Autodesk Fusion 360 part; units mm, degrees
(part 5 of 5)
  spline S9 degree 5 poles (1.8021, -146.297) (1.7927, -146.2963) (1.774, -146.2951) (1.746, -146.2934) (1.7087, -146.2912) (1.6621, -146.2888) (1.6156, -146.2866) (1.5692, -146.2847) (1.5229, -146.2831) (1.4766, -146.2818) (1.4305, -146.2807) (1.3844, -146.2799) (1.3384, -146.2794) (1.2924, -146.2792) (1.2466, -146.2792) (1.2009, -146.2795) (1.1552, -146.2801) (1.1097, -146.281) (1.0642, -146.2822) (1.0189, -146.2836) (0.9736, -146.2854) (0.9285, -146.2874) (0.8834, -146.2897) (0.8385, -146.2923) (0.7937, -146.2951) (0.7489, -146.2983) (0.7044, -146.3018) (0.6599, -146.3055) (0.6155, -146.3095) (0.5713, -146.3139) (0.5271, -146.3185) (0.4832, -146.3234) (0.4393, -146.3287) (0.3956, -146.3342) (0.352, -146.3401) (0.3085, -146.3462) (0.2652, -146.3527) (0.222, -146.3594) (0.179, -146.3665) (0.1361, -146.3739) (0.0934, -146.3816) (0.0508, -146.3896) (0.0084, -146.3979) (-0.0338, -146.4066) (-0.0759, -146.4156) (-0.1178, -146.425) (-0.1596, -146.4346) (-0.2011, -146.4446) (-0.2425, -146.455) (-0.2837, -146.4656) (-0.3247, -146.4767) (-0.3655, -146.4881) (-0.406, -146.4998) (-0.4464, -146.512) (-0.4865, -146.5246) (-0.5264, -146.5375) (-0.5661, -146.5508) (-0.6056, -146.5644) (-0.6449, -146.5784) (-0.6839, -146.5927) (-0.7226, -146.6076) (-0.761, -146.623) (-0.799, -146.639) (-0.8366, -146.6556) (-0.8739, -146.6727) (-0.9109, -146.6902) (-0.9477, -146.708) (-0.9843, -146.726) (-1.0206, -146.7445) (-1.0563, -146.7636) (-1.0913, -146.784) (-1.1184, -146.8016) (-1.138, -146.8156) (-1.1509, -146.8255) (-1.1572, -146.8305) knots -1 -1 -1 -1 -1 -1 -0.98571429 -0.97142857 -0.95714286 -0.94285714 -0.92857143 -0.91428571 -0.9 -0.88571429 -0.87142857 -0.85714286 -0.84285714 -0.82857143 -0.81428571 -0.8 -0.78571429 -0.77142857 -0.75714286 -0.74285714 -0.72857143 -0.71428571 -0.7 -0.68571429 -0.67142857 -0.65714286 -0.64285714 -0.62857143 -0.61428571 -0.6 -0.58571429 -0.57142857 -0.55714286 -0.54285714 -0.52857143 -0.51428571 -0.5 -0.48571429 -0.47142857 -0.45714286 -0.44285714 -0.42857143 -0.41428571 -0.4 -0.38571429 -0.37142857 -0.35714286 -0.34285714 -0.32857143 -0.31428571 -0.3 -0.28571429 -0.27142857 -0.25714286 -0.24285714 -0.22857143 -0.21428571 -0.2 -0.18571429 -0.17142857 -0.15714286 -0.14285714 -0.12857143 -0.11428571 -0.1 -0.08571429 -0.07142857 -0.05714286 -0.04285714 -0.02857143 -0.01428571 0 0 0 0 0 0
  line L9 (-1.1572, -146.8305) -> (-1.7657, -147.3112)
  arc A19 (-3.1074, -147.2186) -> (-1.7657, -147.3112) centre (-2.3856, -146.5265) ccw
  arc A20 (-3.1074, -147.2186) -> (-3.391, -146.935) centre (-10, -153.8276) ccw
  arc A21 (-3.4836, -145.5934) -> (-3.391, -146.935) centre (-2.6989, -146.2132) ccw
  line L10 (-3.4836, -145.5934) -> (-3.0028, -144.9848)
  spline S10 degree 5 poles (-3.0028, -144.9848) (-2.9978, -144.9785) (-2.988, -144.9657) (-2.9739, -144.946) (-2.9564, -144.9189) (-2.936, -144.884) (-2.9169, -144.8482) (-2.8984, -144.8119) (-2.8804, -144.7753) (-2.8626, -144.7385) (-2.8451, -144.7015) (-2.828, -144.6642) (-2.8114, -144.6266) (-2.7954, -144.5886) (-2.78, -144.5502) (-2.7651, -144.5115) (-2.7508, -144.4725) (-2.7368, -144.4332) (-2.7232, -144.3937) (-2.7099, -144.354) (-2.697, -144.3141) (-2.6844, -144.274) (-2.6722, -144.2337) (-2.6604, -144.1931) (-2.649, -144.1523) (-2.638, -144.1113) (-2.6273, -144.0701) (-2.617, -144.0287) (-2.607, -143.9872) (-2.5973, -143.9454) (-2.588, -143.9035) (-2.579, -143.8615) (-2.5703, -143.8192) (-2.562, -143.7768) (-2.5539, -143.7342) (-2.5462, -143.6915) (-2.5389, -143.6486) (-2.5318, -143.6056) (-2.525, -143.5624) (-2.5186, -143.5191) (-2.5124, -143.4757) (-2.5066, -143.4321) (-2.5011, -143.3883) (-2.4958, -143.3445) (-2.4909, -143.3005) (-2.4863, -143.2564) (-2.4819, -143.2121) (-2.4779, -143.1678) (-2.4741, -143.1233) (-2.4707, -143.0787) (-2.4675, -143.034) (-2.4646, -142.9891) (-2.462, -142.9442) (-2.4597, -142.8992) (-2.4577, -142.854) (-2.456, -142.8088) (-2.4546, -142.7634) (-2.4534, -142.7179) (-2.4525, -142.6724) (-2.4519, -142.6268) (-2.4516, -142.581) (-2.4516, -142.5352) (-2.4518, -142.4893) (-2.4523, -142.4433) (-2.4531, -142.3972) (-2.4542, -142.351) (-2.4555, -142.3047) (-2.4571, -142.2584) (-2.459, -142.212) (-2.4612, -142.1655) (-2.4636, -142.1189) (-2.4658, -142.0816) (-2.4675, -142.0536) (-2.4687, -142.0349) (-2.4693, -142.0255) knots 0 0 0 0 0 0 0.01428571 0.02857143 0.04285714 0.05714286 0.07142857 0.08571429 0.1 0.11428571 0.12857143 0.14285714 0.15714286 0.17142857 0.18571429 0.2 0.21428571 0.22857143 0.24285714 0.25714286 0.27142857 0.28571429 0.3 0.31428571 0.32857143 0.34285714 0.35714286 0.37142857 0.38571429 0.4 0.41428571 0.42857143 0.44285714 0.45714286 0.47142857 0.48571429 0.5 0.51428571 0.52857143 0.54285714 0.55714286 0.57142857 0.58571429 0.6 0.61428571 0.62857143 0.64285714 0.65714286 0.67142857 0.68571429 0.7 0.71428571 0.72857143 0.74285714 0.75714286 0.77142857 0.78571429 0.8 0.81428571 0.82857143 0.84285714 0.85714286 0.87142857 0.88571429 0.9 0.91428571 0.92857143 0.94285714 0.95714286 0.97142857 0.98571429 1 1 1 1 1 1
  arc A22 (-2.4693, -142.0255) -> (-3.5444, -141.4048) centre (-10, -153.8276) ccw
  spline S11 degree 5 poles (-3.5444, -141.4048) (-3.5528, -141.409) (-3.5696, -141.4173) (-3.5948, -141.4298) (-3.6282, -141.4466) (-3.6697, -141.4677) (-3.7111, -141.4891) (-3.7522, -141.5107) (-3.7931, -141.5324) (-3.8339, -141.5544) (-3.8744, -141.5766) (-3.9147, -141.5989) (-3.9548, -141.6215) (-3.9947, -141.6443) (-4.0344, -141.6672) (-4.0738, -141.6904) (-4.113, -141.7137) (-4.152, -141.7372) (-4.1908, -141.761) (-4.2294, -141.7849) (-4.2677, -141.809) (-4.3058, -141.8333) (-4.3437, -141.8578) (-4.3813, -141.8826) (-4.4187, -141.9075) (-4.4558, -141.9326) (-4.4927, -141.9579) (-4.5293, -141.9833) (-4.5657, -142.009) (-4.6019, -142.0349) (-4.6378, -142.061) (-4.6734, -142.0872) (-4.7088, -142.1137) (-4.7439, -142.1404) (-4.7787, -142.1672) (-4.8133, -142.1943) (-4.8476, -142.2215) (-4.8816, -142.249) (-4.9153, -142.2766) (-4.9488, -142.3044) (-4.9819, -142.3325) (-5.0148, -142.3607) (-5.0473, -142.3891) (-5.0796, -142.4178) (-5.1115, -142.4466) (-5.1431, -142.4756) (-5.1744, -142.5049) (-5.2054, -142.5343) (-5.2361, -142.564) (-5.2664, -142.5938) (-5.2964, -142.6238) (-5.326, -142.6541) (-5.3553, -142.6846) (-5.3841, -142.7153) (-5.4126, -142.7463) (-5.4407, -142.7774) (-5.4684, -142.8088) (-5.4958, -142.8403) (-5.5228, -142.872) (-5.5495, -142.904) (-5.5756, -142.9362) (-5.6011, -142.9687) (-5.626, -143.0016) (-5.6503, -143.0348) (-5.674, -143.0682) (-5.6973, -143.1019) (-5.7203, -143.1357) (-5.7429, -143.1696) (-5.7651, -143.2037) (-5.7866, -143.2382) (-5.8067, -143.2733) (-5.8213, -143.3021) (-5.8313, -143.3241) (-5.8375, -143.339) (-5.8405, -143.3465) knots -1 -1 -1 -1 -1 -1 -0.98571429 -0.97142857 -0.95714286 -0.94285714 -0.92857143 -0.91428571 -0.9 -0.88571429 -0.87142857 -0.85714286 -0.84285714 -0.82857143 -0.81428571 -0.8 -0.78571429 -0.77142857 -0.75714286 -0.74285714 -0.72857143 -0.71428571 -0.7 -0.68571429 -0.67142857 -0.65714286 -0.64285714 -0.62857143 -0.61428571 -0.6 -0.58571429 -0.57142857 -0.55714286 -0.54285714 -0.52857143 -0.51428571 -0.5 -0.48571429 -0.47142857 -0.45714286 -0.44285714 -0.42857143 -0.41428571 -0.4 -0.38571429 -0.37142857 -0.35714286 -0.34285714 -0.32857143 -0.31428571 -0.3 -0.28571429 -0.27142857 -0.25714286 -0.24285714 -0.22857143 -0.21428571 -0.2 -0.18571429 -0.17142857 -0.15714286 -0.14285714 -0.12857143 -0.11428571 -0.1 -0.08571429 -0.07142857 -0.05714286 -0.04285714 -0.02857143 -0.01428571 0 0 0 0 0 0
  line L11 (-5.8405, -143.3465) -> (-6.1271, -144.0671)
  arc A23 (-7.3354, -144.6577) -> (-6.1271, -144.0671) centre (-7.0563, -143.6974) ccw
  arc A24 (-7.3354, -144.6577) -> (-7.7227, -144.5539) centre (-10, -153.8276) ccw
  arc A25 (-8.4737, -143.4383) -> (-7.7227, -144.5539) centre (-7.4842, -143.5828) ccw
  line L12 (-8.4737, -143.4383) -> (-8.3617, -142.671)
  spline S12 degree 5 poles (-8.3617, -142.671) (-8.3605, -142.663) (-8.3584, -142.6469) (-8.3561, -142.6229) (-8.3544, -142.5906) (-8.3542, -142.5502) (-8.3555, -142.5096) (-8.3577, -142.469) (-8.3604, -142.4282) (-8.3634, -142.3875) (-8.3667, -142.3467) (-8.3705, -142.3059) (-8.375, -142.265) (-8.3801, -142.2241) (-8.386, -142.1832) (-8.3925, -142.1422) (-8.3995, -142.1012) (-8.4071, -142.0602) (-8.415, -142.0192) (-8.4234, -141.9782) (-8.4322, -141.9372) (-8.4413, -141.8961) (-8.4509, -141.8551) (-8.461, -141.8141) (-8.4715, -141.7731) (-8.4825, -141.7321) (-8.4938, -141.691) (-8.5056, -141.65) (-8.5177, -141.6091) (-8.5302, -141.5681) (-8.5431, -141.5271) (-8.5563, -141.4862) (-8.5699, -141.4453) (-8.5839, -141.4044) (-8.5982, -141.3635) (-8.6129, -141.3226) (-8.628, -141.2818) (-8.6434, -141.241) (-8.6591, -141.2002) (-8.6752, -141.1595) (-8.6916, -141.1188) (-8.7083, -141.0781) (-8.7254, -141.0375) (-8.7428, -140.9969) (-8.7605, -140.9563) (-8.7785, -140.9158) (-8.7969, -140.8753) (-8.8156, -140.8348) (-8.8346, -140.7944) (-8.8539, -140.7541) (-8.8735, -140.7138) (-8.8934, -140.6735) (-8.9137, -140.6333) (-8.9342, -140.5932) (-8.955, -140.5531) (-8.9761, -140.513) (-8.9976, -140.473) (-9.0193, -140.4331) (-9.0413, -140.3932) (-9.0636, -140.3533) (-9.0862, -140.3136) (-9.1091, -140.2739) (-9.1322, -140.2342) (-9.1557, -140.1946) (-9.1794, -140.1551) (-9.2034, -140.1156) (-9.2277, -140.0763) (-9.2523, -140.0369) (-9.2771, -139.9977) (-9.3022, -139.9585) (-9.3276, -139.9194) (-9.3482, -139.8881) (-9.3637, -139.8648) (-9.3741, -139.8492) (-9.3793, -139.8414) knots 0 0 0 0 0 0 0.01428571 0.02857143 0.04285714 0.05714286 0.07142857 0.08571429 0.1 0.11428571 0.12857143 0.14285714 0.15714286 0.17142857 0.18571429 0.2 0.21428571 0.22857143 0.24285714 0.25714286 0.27142857 0.28571429 0.3 0.31428571 0.32857143 0.34285714 0.35714286 0.37142857 0.38571429 0.4 0.41428571 0.42857143 0.44285714 0.45714286 0.47142857 0.48571429 0.5 0.51428571 0.52857143 0.54285714 0.55714286 0.57142857 0.58571429 0.6 0.61428571 0.62857143 0.64285714 0.65714286 0.67142857 0.68571429 0.7 0.71428571 0.72857143 0.74285714 0.75714286 0.77142857 0.78571429 0.8 0.81428571 0.82857143 0.84285714 0.85714286 0.87142857 0.88571429 0.9 0.91428571 0.92857143 0.94285714 0.95714286 0.97142857 0.98571429 1 1 1 1 1 1
  arc A26 (-9.3793, -139.8414) -> (-10.6207, -139.8414) centre (-10, -153.8276) ccw
  spline S13 degree 5 poles (-10.6207, -139.8414) (-10.6259, -139.8492) (-10.6363, -139.8648) (-10.6518, -139.8881) (-10.6724, -139.9194) (-10.6978, -139.9585) (-10.7229, -139.9977) (-10.7477, -140.0369) (-10.7723, -140.0763) (-10.7966, -140.1156) (-10.8206, -140.1551) (-10.8443, -140.1946) (-10.8678, -140.2342) (-10.8909, -140.2739) (-10.9138, -140.3136) (-10.9364, -140.3533) (-10.9587, -140.3932) (-10.9807, -140.4331) (-11.0024, -140.473) (-11.0239, -140.513) (-11.045, -140.5531) (-11.0658, -140.5932) (-11.0863, -140.6333) (-11.1066, -140.6735) (-11.1265, -140.7138) (-11.1461, -140.7541) (-11.1654, -140.7944) (-11.1844, -140.8348) (-11.2031, -140.8753) (-11.2215, -140.9158) (-11.2395, -140.9563) (-11.2572, -140.9969) (-11.2746, -141.0375) (-11.2917, -141.0781) (-11.3084, -141.1188) (-11.3248, -141.1595) (-11.3409, -141.2002) (-11.3566, -141.241) (-11.372, -141.2818) (-11.3871, -141.3226) (-11.4018, -141.3635) (-11.4161, -141.4044) (-11.4301, -141.4453) (-11.4437, -141.4862) (-11.4569, -141.5271) (-11.4698, -141.5681) (-11.4823, -141.6091) (-11.4944, -141.65) (-11.5062, -141.691) (-11.5175, -141.7321) (-11.5285, -141.7731) (-11.539, -141.8141) (-11.5491, -141.8551) (-11.5587, -141.8961) (-11.5678, -141.9372) (-11.5766, -141.9782) (-11.585, -142.0192) (-11.5929, -142.0602) (-11.6005, -142.1012) (-11.6075, -142.1422) (-11.614, -142.1832) (-11.6199, -142.2241) (-11.625, -142.265) (-11.6295, -142.3059) (-11.6333, -142.3467) (-11.6366, -142.3875) (-11.6396, -142.4282) (-11.6423, -142.469) (-11.6445, -142.5096) (-11.6458, -142.5502) (-11.6456, -142.5906) (-11.6439, -142.6229) (-11.6416, -142.6469) (-11.6395, -142.663) (-11.6383, -142.671) knots -1 -1 -1 -1 -1 -1 -0.98571429 -0.97142857 -0.95714286 -0.94285714 -0.92857143 -0.91428571 -0.9 -0.88571429 -0.87142857 -0.85714286 -0.84285714 -0.82857143 -0.81428571 -0.8 -0.78571429 -0.77142857 -0.75714286 -0.74285714 -0.72857143 -0.71428571 -0.7 -0.68571429 -0.67142857 -0.65714286 -0.64285714 -0.62857143 -0.61428571 -0.6 -0.58571429 -0.57142857 -0.55714286 -0.54285714 -0.52857143 -0.51428571 -0.5 -0.48571429 -0.47142857 -0.45714286 -0.44285714 -0.42857143 -0.41428571 -0.4 -0.38571429 -0.37142857 -0.35714286 -0.34285714 -0.32857143 -0.31428571 -0.3 -0.28571429 -0.27142857 -0.25714286 -0.24285714 -0.22857143 -0.21428571 -0.2 -0.18571429 -0.17142857 -0.15714286 -0.14285714 -0.12857143 -0.11428571 -0.1 -0.08571429 -0.07142857 -0.05714286 -0.04285714 -0.02857143 -0.01428571 0 0 0 0 0 0
  line L13 (-11.6383, -142.671) -> (-11.5263, -143.4383)
  arc A27 (-12.2773, -144.5539) -> (-11.5263, -143.4383) centre (-12.5158, -143.5828) ccw
  circle A28 centre (-10, -153.8276) radius 2.5
  line L14 (-10, -153.8276) -> (-34.2462, -158.1029)
  line L15 (-10, -153.8276) -> (15, -153.8276) construction
  line L16 (-10, -153.8276) -> (-34.2462, -149.5524)
  line L17 (-10, -153.8276) -> (15, -153.8276) construction
  circle A29 centre (-35, -153.8276) radius 4.3412
  circle A30 centre (-35, -153.8276) radius 2
  circle A31 centre (-10, -153.8276) radius 9.5492
  dimension "d11" = 170
  dimension "d13" = 170
  dimension "d15" = 4
  dimension "d20" = 25
  constraint horizontal L15
  constraint coincident A0.centre A2.centre
  constraint horizontal L17
  constraint coincident L16.end A29
  constraint coincident L14.end A29
  constraint concentric A29 A30
  measures "d11" angle of L14 L15
  measures "d13" angle of L16 L17
  measures "d15" diameter of A30
  measures "d20" distance of A0.centre A29.centre
extrude "Extrude4" add sketch "Sketch2 (2)" against normal blind 5 contours A0 L14 L16 A29 A31 | A29 sketch seen with x (0.979925, -0.165191, 0.111619) y (0.179467, 0.974729, -0.133022) z (-0.086824, 0.150384, 0.984808) at (-68.2536, 138.2186, 733.0373) in component "Spur Gear (12 teeth)"
fillet "Fillet2" radius 5 2 edges at (-8.9733, -3.266, 2.5) (-7.3151, -6.1381, 2.5) in component "Spur Gear (12 teeth)"
component "Spur Gear (12 teeth)" placed x (1, 0, 0) y (0, 1, 0) z (0, 0, 1) at (0, 0, 0)
